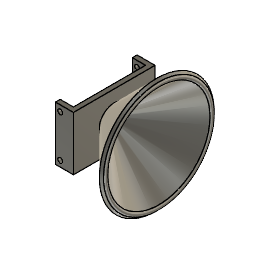
Female Connector (Autodesk Fusion 360 design; units mm, degrees)
Autodesk Fusion 360 part; units mm, degrees
note: some values were not read from the file. Set by a fixed rule: which sketch regions a step uses.
sketch "Sketch1" plane through (0, 0, 0) normal (0, 1, 0) x (1, 0, 0)
  line L0 (7.5, -22.5) -> (-7.5, -22.5)
  line L1 (-7.5, -22.5) -> (-7.5, 22.5)
  line L2 (-7.5, 22.5) -> (7.5, 22.5)
  line L3 (7.5, 22.5) -> (7.5, -22.5)
  line L4 (7.5, -22.5) -> (-7.5, 22.5) construction
  line L5 (-7.5, -22.5) -> (7.5, 22.5) construction
  dimension "d1" = 45
  dimension "d2" = 15
  constraint horizontal L0
  constraint perpendicular L0 L1
  constraint parallel L0 L2
  constraint parallel L1 L3
  constraint coincident L4 origin
  constraint coincident L5 origin
  measures "d1" distance of L0.end L1.end
  measures "d2" distance of L0.start L0.end
extrude "Extrude1" add sketch "Sketch1" along normal blind 4
sketch "Sketch2" plane through (0, 4, 0) normal (0, 1, 0) x (-1, 0, 0)
  line L0 (-7.5, -22.5) -> (7.5, -22.5)
  line L1 (7.5, -22.5) -> (7.5, 22.5)
  line L2 (7.5, 22.5) -> (-7.5, 22.5)
  line L3 (-7.5, 22.5) -> (-7.5, -22.5)
  line L4 (-7.5, 22.5) -> (-3.5, 22.5)
  line L5 (-3.5, 22.5) -> (-3.5, -22.5)
  line L6 (-3.5, -22.5) -> (-7.5, -22.5)
  line L7 (-7.5, -22.5) -> (-7.5, 22.5)
  dimension "d9" = 4
  constraint horizontal L4
  constraint vertical L5
  constraint horizontal L6
  constraint vertical L7
  constraint coincident L0 L5.end
  constraint coincident L2.end L3.start
  measures "d9" distance of L2.end L4.end
extrude "Extrude2" add sketch "Sketch2" along normal blind 64 contours L0 L2 L3 L4 L5 L6 L7
sketch "Sketch3" plane through (3.5, 0, 0) normal (-1, 0, 0) x (0, -1, 0)
  line L0 (-4, -22.5) -> (-4, 22.5)
  line L1 (-4, 22.5) -> (-68, 22.5)
  line L2 (-68, 22.5) -> (-68, -22.5)
  line L3 (-68, -22.5) -> (-4, -22.5)
  line L4 (-68, 22.5) -> (-64, 22.5)
  line L5 (-64, 22.5) -> (-64, -22.5)
  line L6 (-64, -22.5) -> (-68, -22.5)
  line L7 (-68, -22.5) -> (-68, 22.5)
  dimension "d12" = 4
  constraint horizontal L4
  constraint vertical L5
  constraint horizontal L6
  constraint vertical L7
  constraint coincident L3 L5.end
  constraint coincident L1.end L2.start
  measures "d12" distance of L1.end L4.end
extrude "Extrude3" add sketch "Sketch3" along normal blind 11 contours L1 L2 L3 L4 L5 L6 L7
sketch "Sketch4" plane through (3.5, 0, 0) normal (-1, 0, 0) x (0, -1, 0)
  line L0 (-64, 22.5) -> (-64, -22.5)
  line L1 (-64, -22.5) -> (-4, -22.5)
  line L2 (-4, -22.5) -> (-4, 22.5)
  line L3 (-4, 22.5) -> (-64, 22.5)
  line L4 (-60, 22.5) -> (-56, 22.5)
  line L5 (-56, 22.5) -> (-56, -22.5)
  line L6 (-56, -22.5) -> (-60, -22.5)
  line L7 (-60, -22.5) -> (-60, 22.5)
  line L8 (-34, -22.5) -> (-34, 22.5) construction
  line L9 (-8, 22.5) -> (-12, 22.5)
  line L10 (-8, -22.5) -> (-8, 22.5)
  line L11 (-12, 22.5) -> (-12, -22.5)
  line L12 (-12, -22.5) -> (-8, -22.5)
  dimension "d15" = 4
  dimension "d16" = 4
  constraint horizontal L4
  constraint vertical L5
  constraint horizontal L6
  constraint vertical L7
  constraint coincident L1 L5.end
  constraint coincident L3 L4.start
  constraint midpoint L1 L8.start
  constraint midpoint L3 L8.end
  constraint symmetric L4.start L8 L9.start
  constraint symmetric L4.end L8 L9.end
  constraint symmetric L5.end L8 L11.end
  constraint symmetric L6.end L8 L10.start
  measures "d15" distance of L5.end L6.end
  measures "d16" distance of L0 L7
sketch "Sketch5" plane through (0, 68, 0) normal (0, 1, 0) x (-1, 0, 0)
  line L0 (-7.5, -22.5) -> (7.5, -22.5)
  line L1 (7.5, -22.5) -> (7.5, 22.5)
  line L2 (7.5, 22.5) -> (-7.5, 22.5)
  line L3 (-7.5, 22.5) -> (-7.5, -22.5)
  circle A0 centre (3.5, 17.4201) radius 2
  circle A1 centre (3.5, -17.5799) radius 2
  line L4 (3.5, -17.5799) -> (3.5, 17.4201) construction
  point P0 (3.5, -0.0799)
  dimension "d19" = 4
  dimension "d20" = 4
  dimension "d21" = 35
  dimension "d22" = 4
  constraint midpoint L4 P0
  constraint vertical L4
  constraint coincident A0.centre L4.end
  constraint coincident A1.centre L4.start
  measures "d19" diameter of A0
  measures "d20" diameter of A1
  measures "d21" distance of A1.centre A0.centre
  measures "d22" distance of L1 L4
extrude "Extrude5" cut sketch "Sketch5" against normal through all contours A0 | A1
ref_plane "WorkPlane1" through (0, 34, 0) normal (0, 1, 0) x (0, 0, 1)
sketch "Sketch6" plane through (0, 34, 0) normal (0, 1, 0) x (1, 0, 0)
  line L0 (7.5, -12.5) -> (42.8553, -47.8553)
  line L1 (7.5, 22.5) -> (7.5, -22.5)
  line L2 (7.5, 12.5) -> (7.5, -12.5) construction
  line L3 (7.5, 0) -> (0, 0)
  line L4 (42.8553, -47.8553) -> (44.6231, -46.0876)
  line L5 (44.6231, -42.552) -> (7.5, -5.4289)
  arc A0 (44.6231, -46.0876) -> (44.6231, -42.552) centre (42.8553, -44.3198) ccw
  point P0 (7.5, 0)
  point P1 (46.3909, -44.3198)
  dimension "d25" = 50
  dimension "d26" = 25
  dimension "d27" = 135
  dimension "d29" = 5
  dimension "d30" = 2.5
  constraint coincident L0.start L1
  constraint midpoint L2 P0
  constraint coincident L1 P0
  constraint parallel L1 L2
  constraint coincident L0.start L2.end
  constraint coincident P0 L3.start
  constraint coincident L3.end origin
  constraint horizontal L3
  constraint perpendicular L0 L4
  constraint coincident L2 L5.end
  constraint parallel L0 L5
  constraint coincident P1 L5
  constraint coincident P1 L4
  constraint tangent L5 A0
  constraint tangent L4 A0
  measures "d25" distance of L0.start L0.end
  measures "d26" distance of L2.start L0.start
  measures "d27" angle of L0 L2
  measures "d29" distance of L0.end P1
  measures "d30" radius of A0
revolve "Revolve1" add sketch "Sketch6" angle 360 about axis through (7.5, 34, 0) along (-1, 0, 0)
equation "d10 = 56 mm + 8 mm"
equation "d24 = -( 68 / 2 ) * 1 mm"
